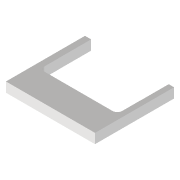
# Autodesk Inventor part: 30_XYTable_Aliexpress_CAM_cutout
Saved by Autodesk Inventor 2022 (Build 260153000, 153)
## iProperties
Created: 2022-10-14
Part Number: 30_XYTable_Aliexpress_CAM_cutout
Material: Generisch
Document SubType Name: Modeling
Designer: diederichbenedict
Density: 1 g/cm^3
Appearance: Vorgabe
Author: diederichbenedict
Autodesk Inventor part; units mm, degrees
ref_plane "YZ Plane" through (0, 0, 0) normal (1, 0, 0) x (0, 1, 0)
ref_plane "XZ Plane" through (0, 0, 0) normal (0, 1, 0) x (-1, 0, 0)
ref_plane "XY Plane" through (0, 0, 0) normal (0, 0, 1) x (1, 0, 0)
sketch "Skizze1" plane through (0, 0, 0) normal (0, 1, 0) x (-1, 0, 0)
  line L0 (0, 0) -> (-109.21, 0)
  line L1 (-109.21, 0) -> (-109.21, 96.9)
  line L2 (-109.21, 96.9) -> (0, 96.9)
  line L3 (0, 96.9) -> (0, 0)
  dimension "d5" = 109.21
  dimension "d6" = 96.9
  constraints: 8 end point, 2 parallel, 1 horizontal, 1 perpendicular
  measures "d5" distance between parallel lines of L1 L3
  measures "d6" distance between parallel lines of L0 L2
extrude "Extrusion1" add sketch "Skizze1" along normal blind 12
sketch "Skizze2" plane through (0, 12, 0) normal (0, 1, 0) x (1, 0, 0)
  line L0 (7.6, 0) -> (102.6, 0)
  line L1 (102.6, 0) -> (102.6, -56.9)
  line L2 (96.6, -62.9) -> (13.6, -62.9)
  line L3 (7.6, -56.9) -> (7.6, 0)
  arc A0 (7.6, -56.9) -> (13.6, -62.9) centre (13.6, -56.9) ccw
  arc A1 (96.6, -62.9) -> (102.6, -56.9) centre (96.6, -56.9) ccw
  line L4 (0, 0) -> (0, -96.9) projected
  line L5 (109.21, 0) -> (0, 0) projected
  dimension "d2" = 6
  dimension "d7" = 7.6
  dimension "d8" = 62.9
  dimension "d9" = 95
  constraints: 8 end point, 4 point on circle, 4 tangent, 2 centre point, 2 parallel, 1 equal radius, 1 horizontal, 1 perpendicular, 1 point on line
  measures "d2" radius of A0
  measures "d7" distance between parallel lines of L3 L4
  measures "d8" distance between parallel lines of L2 L0
  measures "d9" distance between parallel lines of L1 L3
extrude "Extrusion2" cut sketch "Skizze2" against normal through all
sketch "Skizze3" plane through (0, 12, 0) normal (0, 1, 0) x (1, 0, 0)
  line L0 (7.6, -56.9) -> (7.6, 0) projected
  line L1 (7.6, 0) -> (0, 0) projected
  line L2 (0, 0) -> (0, -96.9) projected
  line L3 (0, -96.9) -> (109.21, -96.9) projected
  line L4 (109.21, -96.9) -> (109.21, 0) projected
  line L5 (109.21, 0) -> (102.6, 0) projected
  line L6 (102.6, 0) -> (102.6, -56.9) projected
  arc A0 (96.6, -62.9) -> (102.6, -56.9) centre (96.6, -56.9) ccw projected
  line L7 (96.6, -62.9) -> (13.6, -62.9) projected
  arc A1 (7.6, -56.9) -> (13.6, -62.9) centre (13.6, -56.9) ccw projected
  line L8 (102.6, 0) -> (102.7, 0)
  line L9 (102.7, 0) -> (102.7, -35)
  line L10 (102.7, -35) -> (102.6, -35)
  line L11 (102.6, -35) -> (102.6, 0)
  line L12 (7.6, 0) -> (7.6, -56.9) projected
  line L13 (7.6, 0) -> (7.5, 0)
  line L14 (7.5, 0) -> (7.5, -40)
  line L15 (7.5, -40) -> (7.6, -40)
  line L16 (7.6, -40) -> (7.6, 0)
  point P0 (102.6, -35)
  dimension "d10" = 0.1
  dimension "d11" = 35
  dimension "d12" = 0.1
  constraints: 16 end point, 4 parallel, 2 horizontal, 2 perpendicular
  measures "d10" distance of L9.end L10.end
  measures "d11" distance from line of L5 L10.end
  measures "d12" distance of L15.end L14.end
extrude "Extrusion3" cut sketch "Skizze3" against normal through all contours L15 L14 L1 L0 | L6 L5 L9 L10
